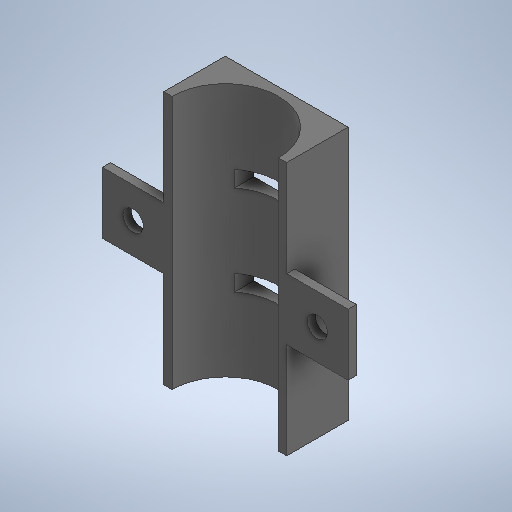
# Autodesk Inventor part: Motorhalterung_Teil2
Saved by Autodesk Inventor 2025.1 (Build 291241000, 241)
## iProperties
Created: 2024-12-18
Part Number: Motorhalterung_Teil2
Material: Generisch
Document SubType Name: Modeling
Designer: Julian
Density: 1 g/cm^3
Appearance: Vorgabe
Author: Julian
Autodesk Inventor part; units mm, degrees
ref_plane "YZ Plane" through (0, 0, 0) normal (1, 0, 0) x (0, 1, 0)
ref_plane "XZ Plane" through (0, 0, 0) normal (0, 1, 0) x (-1, 0, 0)
ref_plane "XY Plane" through (0, 0, 0) normal (0, 0, 1) x (1, 0, 0)
sketch "Skizze4" plane through (0, 0, 0) normal (0, 0, 1) x (1, 0, 0)
  line L0 (15, 15) -> (-15, 15)
  line L1 (-15, 15) -> (-15, 0)
  line L2 (-15, -15) -> (15, 15) construction
  line L3 (15, -15) -> (-15, 15) construction
  line L4 (-15, 0) -> (15, 0)
  arc A0 (13, 0) -> (-13, 0) centre (0, 0) ccw
  line L5 (15, 0) -> (15, 15)
  dimension "d9" = 30
  dimension "d10" = 30
  constraints: 12 end point, 2 midpoint, 2 point on circle, 2 point on line, 1 centre point, 1 coincident, 1 vertical
  measures "d9" distance of L0.end L0.start
  measures "d10" distance of L0.start L3.start
extrude "Extrusion4" add sketch "Skizze4" along normal blind 30 contours L5 L4 A0 L1 L0
sketch "Skizze5" plane through (0, 0, 0) normal (0, 0, -1) x (-1, 0, 0)
  line L0 (-15, 0) -> (-15, 15) projected
  line L1 (15, 0) -> (13, 0) projected
  line L2 (-15, 15) -> (15, 15)
  line L3 (15, 15) -> (15, 0)
  line L4 (15, 0) -> (-15, 0)
  line L5 (-15, 0) -> (-15, 15)
  point P0 (0, 0)
  constraints: 8 end point, 2 parallel, 1 horizontal, 1 perpendicular
extrude "Extrusion5" add sketch "Skizze5" along normal blind 2
sketch "Skizze6" plane through (0, 0, -2) normal (0, 0, -1) x (-1, 0, 0)
  line L0 (-15, 0) -> (-15, 15) projected
  line L1 (15, 0) -> (13, 0) projected
  line L2 (-15, 15) -> (15, 15)
  line L3 (15, 15) -> (15, 0)
  line L4 (15, 0) -> (-15, 0)
  line L5 (-15, 0) -> (-15, 15)
  arc A0 (13, 0) -> (-13, 0) centre (0, 0) ccw
  dimension "d16" = 26
  constraints: 8 end point, 2 parallel, 2 point on circle, 2 point on line, 1 centre point, 1 coincident, 1 horizontal, 1 perpendicular
  measures "d16" diameter of A0
extrude "Extrusion6" add sketch "Skizze6" along normal blind 30 contours L0 L2 L3 L1 A0 L4
sketch "Skizze9" plane through (15, 0, 30) normal (1, 0, 0) x (0, 0, -1)
  line L0 (0, 0) -> (0, 13) projected
  line L1 (62, 13) -> (62, 0) projected
  line L2 (62, 0) -> (0, 0) projected
  line L3 (23.5, 2) -> (38.5, 2)
  line L4 (38.5, 2) -> (38.5, 0)
  line L5 (38.5, 0) -> (23.5, 0)
  line L6 (23.5, 0) -> (23.5, 2)
  line L7 (23.5, 2) -> (38.5, 0) construction
  line L8 (38.5, 2) -> (23.5, 0) construction
  point P0 (30, 0)
  point P1 (31, 1)
  dimension "d36" = 15
  constraints: 12 end point, 2 midpoint, 2 parallel, 1 horizontal, 1 perpendicular, 1 point on line
  measures "d36" distance of L4.end L5.end
extrude "Extrusion8" add sketch "Skizze9" along normal blind 15
sketch "Skizze10" plane through (-15, 0, 30) normal (-1, 0, 0) x (0, 0, 1)
  line L0 (0, 0) -> (0, 15) projected
  line L1 (0, 6.5004) -> (31, 6.5004) construction
  line L2 (0, 0) -> (-62, 0) projected
  line L3 (-31, 0) -> (-31, 1)
  line L4 (-38.5, 2) -> (-23.5, 2)
  line L5 (-23.5, 2) -> (-23.5, 0)
  line L6 (-23.5, 0) -> (-38.5, 0)
  line L7 (-38.5, 0) -> (-38.5, 2)
  line L8 (-38.5, 2) -> (-23.5, 0) construction
  line L9 (-23.5, 2) -> (-38.5, 0) construction
  point P0 (-30, 0)
  dimension "d41" = 1
  dimension "d42" = 15
  dimension "d43" = 2
  constraints: 16 end point, 3 midpoint, 2 horizontal, 2 parallel, 1 perpendicular, 1 point on line
  measures "d41" distance of L3.start L3.end
  measures "d42" distance of L5.end L6.end
  measures "d43" distance of L4.end L5.end
extrude "Extrusion9" add sketch "Skizze10" along normal blind 15
sketch "Skizze11" plane through (-15, 15, 30) normal (0, 1, 0) x (1, 0, 0)
  line L0 (0, 23.5) -> (-15, 23.5) projected
  line L1 (0, 62) -> (0, 0) projected
  line L2 (30, 62) -> (30, 0) projected
  line L3 (23, 22) -> (7, 22)
  line L4 (7, 22) -> (7, 18)
  line L5 (7, 18) -> (23, 18)
  line L6 (23, 18) -> (23, 22)
  line L7 (23, 22) -> (7, 18) construction
  line L8 (7, 22) -> (23, 18) construction
  line L9 (7, 44) -> (23, 44)
  line L10 (23, 44) -> (23, 40)
  line L11 (23, 40) -> (7, 40)
  line L12 (7, 40) -> (7, 44)
  line L13 (7, 44) -> (23, 40) construction
  line L14 (23, 44) -> (7, 40) construction
  point P0 (15, 30)
  dimension "d55" = 16
  dimension "d56" = 4
  dimension "d58" = 16
  dimension "d59" = 4
  constraints: 24 end point, 4 parallel, 2 horizontal, 2 perpendicular
  measures "d55" distance of L5.end L4.end
  measures "d56" distance of L4.end L3.end
  measures "d58" distance of L10.end L11.end
  measures "d59" distance of L9.end L10.end
extrude "Extrusion10" cut sketch "Skizze11" against normal through all
sketch "Skizze12" plane through (-15, 2, 6.5) normal (0, 1, 0) x (1, 0, 0)
  line L0 (-15, 15) -> (-15, 0) projected
  line L1 (0, 38.5) -> (0, -23.5) projected
  line L2 (-15, 0) -> (6.2132, 0) construction
  circle A0 centre (-7.5, 7.5) radius 2.5
  point P0 (15, 6.5)
  dimension "d63" = 5
  constraints: 2 end point, 1 centre point, 1 horizontal
  measures "d63" diameter of A0
extrude "Extrusion11" cut sketch "Skizze12" against normal through all
sketch "Skizze13" plane through (15, 2, 6.5) normal (0, 1, 0) x (1, 0, 0)
  line L0 (0, 0) -> (15, 0) projected
  line L1 (0, 38.5) -> (0, -23.5) projected
  line L2 (15, 0) -> (36.2132, 0) construction
  circle A0 centre (7.5, 7.5) radius 2.5
  point P0 (-15, 6.5)
  dimension "d67" = 5
  constraints: 2 end point, 1 centre point, 1 horizontal
  measures "d67" diameter of A0
extrude "Extrusion12" cut sketch "Skizze13" against normal blind 10
sketch "Skizze15" plane through (0, 0, -2) normal (0, 0, -1) x (-1, 0, 0)
  circle A0 centre (0, 0) radius 13
  constraints: 1 centre point, 1 coincident
extrude "Extrusion14" cut sketch "Skizze15" against normal blind 2
